Autodesk Fusion 360 part; units mm, degrees
note: some values were not read from the file. Set by a fixed rule: which face or edge a step refers to.
(part 5 of 5)
sketch "Sketch4" plane through (0, 3.5, 0) normal (0, 1, 0) x (-1, 0, 0)
  line L0 (71.3671, -5) -> (71.3671, 5)
  line L1 (71.3671, 5) -> (56.3671, 5)
  line L2 (56.3671, 5) -> (56.3671, -5)
  line L3 (56.3671, -5) -> (71.3671, -5)
  circle A0 centre (63.8671, 0) radius 2.125
  line L4 (31.5162, -5) -> (9.7806, -5)
  line L5 (31.5162, 5) -> (31.5162, -5)
  line L6 (9.7806, -5) -> (9.7806, 5)
  dimension "d25" = 4.25
  dimension "d27" = 5
  dimension "d31" = 7.5
  dimension "d32" = 7.5
  measures "d25" diameter of A0
  measures "d27" distance of L3 A0.centre
  measures "d31" distance of L0 A0.centre
  measures "d32" distance of L2 A0.centre
extrude "Extrude4" cut sketch "Sketch4" along normal up to surface contours A0 end surface through (-31.4507, -3.3834, 0) normal (0.009359, -0.999956, 0) offset 0
sketch "Sketch5" plane through (-0.0366, 3.9109, 0) normal (-0.009359, 0.999956, 0) x (0, 0, 1)
  line L0 (-5, -31.481) -> (5, -31.481)
  line L1 (5, -31.481) -> (5, -9.7444)
  line L2 (5, -9.7444) -> (-5, -9.7444)
  line L3 (-5, -9.7444) -> (-5, -31.481)
  circle A0 centre (0, -20.613) radius 2.125
  dimension "d35" = 4.25
  dimension "d36" = 10.868
  dimension "d37" = 10.8686
  dimension "d38" = 5
  measures "d35" diameter of A0
  measures "d36" distance of L0 A0.centre
  measures "d37" distance of L2 A0.centre
  measures "d38" distance of L3 A0.centre
extrude "Extrude5" cut sketch "Sketch5" against normal up to surface (7 mm away) contours A0
sketch "Sketch6" plane through (0, 3.5, 0) normal (0, 1, 0) x (-1, 0, 0)
  line L0 (-9.8995, -5) -> (-9.8995, 5)
  line L1 (-9.8995, 5) -> (-69.8995, 5)
  line L2 (-69.8995, 5) -> (-69.8995, -5)
  line L3 (-69.8995, -5) -> (-9.8995, -5)
sketch "Sketch7" plane through (0, 3.5, 0) normal (0, 1, 0) x (-1, 0, 0)
  line L0 (-9.8995, -5) -> (-9.8995, 5) construction
  line L1 (-9.8995, 5) -> (-69.8995, 5) construction
  line L2 (-69.8995, 5) -> (-69.8995, -5) construction
  line L3 (-69.8995, -5) -> (-9.8995, -5) construction
  line L4 (-69.8995, 0) -> (-9.8995, 0) construction
  circle A0 centre (-61.8995, 0) radius 2.125
  circle A1 centre (-14.8995, 0) radius 2.125
  dimension "d41" = 4.25
  dimension "d42" = 4.25
  dimension "d43" = 8
  dimension "d44" = 5
  constraint midpoint L2 L4.start
  constraint midpoint L0 L4.end
  constraint coincident L4 A0.centre
  constraint coincident L4 A1.centre
  measures "d41" diameter of A0
  measures "d42" diameter of A1
  measures "d43" distance of L2 A0.centre
  measures "d44" distance of L0 A1.centre
extrude "Extrude6" cut sketch "Sketch7" against normal up to surface (7 mm away)
sketch "Sketch10" plane through (0, 0, 5) normal (0, 0, 1) x (1, 0, 0)
  circle A0 centre (0, 0) radius 6.75
  arc A1 (-31.5162, 3.6163) -> (-56.3671, 3.5) centre (-43.925, 0) ccw
  line L0 (-56.3671, 3.5) -> (-71.3671, 3.5)
  line L1 (-71.3671, 3.5) -> (-71.3671, -3.5)
  line L2 (-71.3671, -3.5) -> (-56.3671, -3.5)
  arc A2 (-56.3671, -3.5) -> (-31.4507, -3.3834) centre (-43.925, 0) ccw
  line L3 (-31.4507, -3.3834) -> (-10.006, -3.1827)
  arc A3 (-10.006, -3.1827) -> (9.8995, -3.5) centre (0, 0) ccw
  line L4 (9.8995, -3.5) -> (69.8995, -3.5)
  line L5 (69.8995, -3.5) -> (69.8995, 3.5)
  line L6 (69.8995, 3.5) -> (9.8995, 3.5)
  arc A4 (9.8995, 3.5) -> (-9.7806, 3.8197) centre (0, 0) ccw
  line L7 (-9.7806, 3.8197) -> (-31.5162, 3.6163)
  circle A5 centre (-43.925, 0) radius 12.925 construction
  circle A6 centre (-43.925, 0) radius 10.37
  dimension "d58" = 20.74
  constraint coincident A1.end A5
  constraint coincident L2.end A5
  constraint coincident A1.start A5
  constraint concentric A1 A6
  measures "d58" diameter of A6
sketch "Sketch11" plane through (0, 0, -5) normal (0, 0, -1) x (-1, 0, 0)
  circle A0 centre (0, 0) radius 6.75
  arc A1 (56.3671, 3.5) -> (31.5162, 3.6163) centre (43.925, 0) ccw
  line L0 (31.5162, 3.6163) -> (9.7806, 3.8197)
  arc A2 (9.7806, 3.8197) -> (-9.8995, 3.5) centre (0, 0) ccw
  line L1 (-9.8995, 3.5) -> (-69.8995, 3.5)
  line L2 (-69.8995, 3.5) -> (-69.8995, -3.5)
  line L3 (-69.8995, -3.5) -> (-9.8995, -3.5)
  arc A3 (-9.8995, -3.5) -> (10.006, -3.1827) centre (0, 0) ccw
  line L4 (10.006, -3.1827) -> (31.4507, -3.3834)
  arc A4 (31.4507, -3.3834) -> (56.3671, -3.5) centre (43.925, 0) ccw
  line L5 (56.3671, -3.5) -> (71.3671, -3.5)
  line L6 (71.3671, -3.5) -> (71.3671, 3.5)
  line L7 (71.3671, 3.5) -> (56.3671, 3.5)
  circle A5 centre (43.925, 0) radius 12.925 construction
  circle A6 centre (43.925, 0) radius 10.6
  dimension "d59" = 21.2
  constraint coincident A1.end A5
  constraint coincident L4.end A5
  constraint coincident A1.start A5
  constraint concentric A1 A6
  measures "d59" diameter of A6
loft "Loft1" cut profiles "Sketch10", "Sketch11" section 1 contours A6 section 2 contours A6
sketch "Sketch8" plane through (0, 0, 5) normal (0, 0, 1) x (1, 0, 0)
  line L0 (-71.3671, 3.5) -> (-71.3671, -3.5)
  line L1 (-71.3671, -3.5) -> (-56.3671, -3.5)
  arc A0 (-56.3671, -3.5) -> (-31.4507, -3.3834) centre (-43.925, 0) ccw
  line L2 (-31.4507, -3.3834) -> (-10.006, -3.1827)
  arc A1 (-10.006, -3.1827) -> (9.8995, -3.5) centre (0, 0) ccw
  line L3 (9.8995, -3.5) -> (69.8995, -3.5)
  line L4 (69.8995, -3.5) -> (69.8995, 3.5)
  line L5 (52.6495, 0) -> (52.6495, -28) construction
  line L6 (52.6495, -28) -> (21.6495, -28) construction
  line L7 (21.6495, -28) -> (21.6495, 0) construction
  circle A2 centre (37.1495, -12.5) radius 12.5 construction
  line L8 (37.1495, -12.5) -> (37.1495, 0) construction
  line L9 (37.1495, -12.5) -> (52.6495, -12.5) construction
  line L10 (37.1495, -12.5) -> (21.6495, -12.5) construction
  line L11 (24.6495, -12.5) -> (24.6495, 0)
  line L12 (49.6495, -12.5) -> (49.6495, 0)
  arc A3 (24.6495, -12.5) -> (49.6495, -12.5) centre (37.1495, -12.5) ccw
  arc A4 (21.6495, -12.5) -> (37.1495, -28) centre (37.1495, -12.5) ccw
  arc A5 (37.1495, -28) -> (52.6495, -12.5) centre (37.1495, -12.5) ccw
  line L13 (21.6495, -12.5) -> (21.6495, 0)
  line L14 (52.6495, -12.5) -> (52.6495, 0)
  line L15 (21.6495, 0) -> (52.6495, 0)
  circle A6 centre (-43.925, 0) radius 10.37
  circle A7 centre (0, 0) radius 6.75
  arc A8 (-31.5162, 3.6163) -> (-56.3671, 3.5) centre (-43.925, 0) ccw
  line L16 (-56.3671, 3.5) -> (-71.3671, 3.5)
  line L17 (69.8995, 3.5) -> (9.8995, 3.5)
  arc A9 (9.8995, 3.5) -> (-9.7806, 3.8197) centre (0, 0) ccw
  line L18 (-9.7806, 3.8197) -> (-31.5162, 3.6163)
  point P0 (37.1495, 0)
  dimension "d49" = 17.25
  dimension "d50" = 31
  dimension "d51" = 28
  dimension "d52" = 25
  constraint vertical L5
  constraint horizontal L6
  constraint vertical L7
  constraint coincident A2.centre L8.start
  constraint coincident L8 P0
  constraint coincident A2 P0
  constraint coincident L5 L9.end
  constraint perpendicular L5 L9
  constraint coincident L7 L10.end
  constraint perpendicular L7 L10
  constraint coincident A2 L11.start
  constraint coincident L10 L11.start
  constraint tangent A2 L11
  constraint coincident A2 L12.start
  constraint coincident L9 L12.start
  constraint tangent A2 L12
  constraint tangent L12 A3
  constraint tangent L6 A4
  constraint coincident L6 A4.end
  constraint tangent L5 A5
  constraint perpendicular L14 L15
  constraint coincident L11.end L15
  constraint coincident L12.end L15
  constraint coincident P0 L15
  constraint midpoint P0 L15
  measures "d49" distance of L4 L5
  measures "d50" distance of L7.end L5.start
  measures "d51" distance of L5.start L5.end
  measures "d52" diameter of A2
extrude "Extrude7" add sketch "Sketch8" against normal up to surface (10 mm away) contours L3 L11 L12 A3 A4 A5 L13 L14
sketch "Sketch9" plane through (0, 0, 5) normal (0, 0, 1) x (1, 0, 0)
  line L0 (21.6495, -3.5) -> (21.6495, -12.5)
  arc A0 (21.6495, -12.5) -> (37.1495, -28) centre (37.1495, -12.5) ccw
  line L1 (52.6495, -12.5) -> (52.6495, -3.5)
  line L2 (-71.3671, 3.5) -> (-71.3671, -3.5)
  line L3 (-71.3671, -3.5) -> (-56.3671, -3.5)
  arc A1 (-56.3671, -3.5) -> (-31.4507, -3.3834) centre (-43.925, 0) ccw
  line L4 (-31.4507, -3.3834) -> (-10.006, -3.1827)
  arc A2 (-10.006, -3.1827) -> (9.8995, -3.5) centre (0, 0) ccw
  line L5 (9.8995, -3.5) -> (21.6495, -3.5)
  line L6 (49.6495, -3.5) -> (49.6495, -12.5)
  arc A3 (24.6495, -12.5) -> (49.6495, -12.5) centre (37.1495, -12.5) ccw
  line L7 (24.6495, -12.5) -> (24.6495, -3.5)
  line L8 (24.6495, -3.5) -> (49.6495, -3.5)
  line L9 (24.6495, -3.5) -> (49.6495, -3.5)
  line L10 (49.6495, -3.5) -> (49.6495, 0)
  line L11 (49.6495, 0) -> (24.6495, 0)
  line L12 (24.6495, 0) -> (24.6495, -3.5)
  circle A4 centre (-43.925, 0) radius 10.37
  circle A5 centre (0, 0) radius 6.75
  line L13 (69.8995, 3.5) -> (9.8995, 3.5)
  arc A6 (9.8995, 3.5) -> (-9.7806, 3.8197) centre (0, 0) ccw
  line L14 (-9.7806, 3.8197) -> (-31.5162, 3.6163)
  arc A7 (-31.5162, 3.6163) -> (-56.3671, 3.5) centre (-43.925, 0) ccw
  line L15 (-56.3671, 3.5) -> (-71.3671, 3.5)
  line L16 (0, 0) -> (24.6495, 0) construction
  constraint horizontal L9
  constraint vertical L10
  constraint horizontal L11
  constraint vertical L12
  constraint coincident L7.end L8.start
  constraint coincident L6.start L8.end
  constraint coincident A2.centre A5.centre
  constraint perpendicular L12 L16
extrude "Extrude8" cut sketch "Sketch9" against normal up to surface (10 mm away) contours L8 L9 L10 L11 L12
sketch "Sketch3" plane through (0, 0, 0) normal (0, 1, 0) x (1, 0, 0)
  line L0 (-71.3671, 5) -> (-71.3671, -5)
  line L1 (-71.3671, -5) -> (-56.3671, -5)
  line L2 (-56.3671, -5) -> (-56.3671, 5)
  line L3 (-56.3671, 5) -> (-71.3671, 5)
  line L4 (9.8995, 5) -> (9.8995, -5)
  line L5 (9.8995, -5) -> (69.8995, -5)
  line L6 (69.8995, -5) -> (69.8995, 5)
  line L7 (69.8995, 5) -> (9.8995, 5)
  line L8 (-71.3671, 5) -> (69.8995, 5)
  line L9 (69.8995, 5) -> (69.8995, -5)
  line L10 (69.8995, -5) -> (-71.3671, -5)
  line L11 (-71.3671, -5) -> (-71.3671, 5)
  circle A0 centre (-63.8671, 0) radius 2.125
  circle A1 centre (14.8995, 0) radius 2.125
  circle A2 centre (61.8995, 0) radius 2.125
  constraint horizontal L8
  constraint vertical L9
  constraint horizontal L10
  constraint vertical L11
  constraint coincident L5.end L6.start
  constraint coincident L0.start L3.end
extrude "Extrude3" [rolled back] along distance 20 taper angle 0
equation "d2 = d1"
equation "d3 = d1"
equation "d4 = d1"
equation "d5 = d1"
equation "d6 = d1"
equation "d42 = d41"
equation "d49 = 20.25 mm - 3 mm"
equation "d50 = 25 mm + 6 mm"
equation "d51 = 25 mm + 3 mm"
